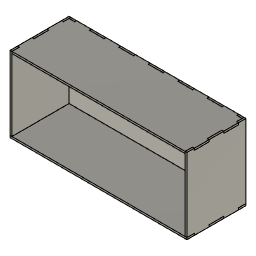
ShockBox 2.0 Enclosure v4 (Autodesk Fusion 360 design; units mm, degrees)
Autodesk Fusion 360 part; units mm, degrees
note: some values were not read from the file. Set by a fixed rule: which sketch regions a step uses.
sketch "Sketch1" plane through (0, 0, 0) normal (0, 1, 0) x (1, 0, 0)
  line L0 (0, 0) -> (304.8, 0)
  line L1 (304.8, 0) -> (304.8, -101.6)
  line L2 (304.8, -101.6) -> (0, -101.6)
  line L3 (0, -101.6) -> (0, 0)
  dimension "d1" = 304.8
  dimension "d2" = 101.6
  constraint horizontal L0
  constraint vertical L1
  constraint horizontal L2
  constraint vertical L3
  constraint coincident L0.start L3.end
  measures "d1" distance of L0.start L0.end
  measures "d2" distance of L0.end L1.end
extrude "Extrude1" add sketch "Sketch1" along normal blind 3.175 makes body 1 in component "Base"
sketch "Sketch2" plane through (0, 0, 0) normal (0, -1, 0) x (1, 0, 0)
  line L0 (304.8, 101.6) -> (0, 101.6)
  line L1 (0, 101.6) -> (0, 0)
  line L2 (0, 0) -> (304.8, 0)
  line L3 (304.8, 0) -> (304.8, 101.6)
  line L4 (0, 101.6) -> (0, 88.9)
  line L5 (0, 88.9) -> (3.175, 88.9)
  line L6 (3.175, 88.9) -> (3.175, 63.5)
  line L7 (3.175, 63.5) -> (0, 63.5)
  line L8 (0, 88.9) -> (0, 63.5)
  line L9 (0, 63.5) -> (0, 38.1)
  line L10 (0, 38.1) -> (3.175, 38.1)
  line L11 (3.175, 38.1) -> (3.175, 12.7)
  line L12 (3.175, 12.7) -> (0, 12.7)
  line L13 (0, 38.1) -> (0, 12.7)
  line L14 (0, 101.6) -> (12.7, 101.6)
  line L15 (12.7, 101.6) -> (12.7, 98.425)
  line L16 (12.7, 98.425) -> (38.1, 98.425)
  line L17 (38.1, 98.425) -> (38.1, 101.6)
  line L18 (38.1, 101.6) -> (12.7, 101.6)
  line L19 (38.1, 101.6) -> (63.5, 101.6)
  line L20 (63.5, 101.6) -> (63.5, 98.425)
  line L21 (63.5, 98.425) -> (88.9, 98.425)
  line L22 (88.9, 98.425) -> (88.9, 101.6)
  line L23 (88.9, 101.6) -> (63.5, 101.6)
  line L24 (88.9, 101.6) -> (114.3, 101.6)
  line L25 (114.3, 101.6) -> (114.3, 98.425)
  line L26 (114.3, 98.425) -> (139.7, 98.425)
  line L27 (139.7, 98.425) -> (139.7, 101.6)
  line L28 (139.7, 101.6) -> (114.3, 101.6)
  line L29 (139.7, 101.6) -> (165.1, 101.6)
  line L30 (165.1, 101.6) -> (165.1, 98.425)
  line L31 (165.1, 98.425) -> (190.5, 98.425)
  line L32 (190.5, 98.425) -> (190.5, 101.6)
  line L33 (190.5, 101.6) -> (165.1, 101.6)
  line L34 (190.5, 101.6) -> (215.9, 101.6)
  line L35 (215.9, 101.6) -> (215.9, 98.425)
  line L36 (215.9, 98.425) -> (241.3, 98.425)
  line L37 (241.3, 98.425) -> (241.3, 101.6)
  line L38 (215.9, 101.6) -> (241.3, 101.6)
  line L39 (241.3, 101.6) -> (266.7, 101.6)
  line L40 (266.7, 101.6) -> (266.7, 98.425)
  line L41 (266.7, 98.425) -> (292.1, 98.425)
  line L42 (292.1, 98.425) -> (292.1, 101.6)
  line L43 (292.1, 101.6) -> (266.7, 101.6)
  line L44 (304.8, 101.6) -> (304.8, 88.9)
  line L45 (304.8, 88.9) -> (301.625, 88.9)
  line L46 (301.625, 88.9) -> (301.625, 63.5)
  line L47 (301.625, 63.5) -> (304.8, 63.5)
  line L48 (304.8, 63.5) -> (304.8, 38.1)
  line L49 (304.8, 38.1) -> (301.625, 38.1)
  line L50 (301.625, 38.1) -> (301.625, 12.7)
  line L51 (301.625, 12.7) -> (304.8, 12.7)
  line L52 (304.8, 12.7) -> (304.8, 38.1)
  line L53 (304.8, 63.5) -> (304.8, 88.9)
  dimension "d7" = 12.7
  dimension "d8" = 3.175
  dimension "d9" = 25.4
  dimension "d10" = 25.4
  dimension "d11" = 3.175
  dimension "d12" = 25.4
  dimension "d13" = 12.7
  dimension "d14" = 3.175
  dimension "d15" = 25.4
  dimension "d16" = 25.4
  dimension "d17" = 3.175
  dimension "d18" = 25.4
  dimension "d19" = 25.4
  dimension "d20" = 3.175
  dimension "d21" = 25.4
  dimension "d22" = 25.4
  dimension "d23" = 3.175
  dimension "d24" = 25.4
  dimension "d25" = 25.4
  dimension "d26" = 25.4
  dimension "d27" = 25.4
  dimension "d28" = 25.4
  dimension "d29" = 12.7
  dimension "d30" = 3.175
  dimension "d31" = 25.4
  dimension "d32" = 25.4
  dimension "d33" = 3.175
  dimension "d34" = 25.4
  constraint coincident L0.end L1.start
  constraint perpendicular L0 L4
  constraint perpendicular L1 L5
  constraint perpendicular L5 L6
  constraint coincident L1 L7.end
  constraint perpendicular L1 L7
  constraint perpendicular L7 L9
  constraint perpendicular L1 L10
  constraint perpendicular L10 L11
  constraint coincident L1 L12.end
  constraint perpendicular L1 L12
  constraint perpendicular L4 L14
  constraint perpendicular L14 L15
  constraint perpendicular L15 L16
  constraint coincident L0 L17.end
  constraint perpendicular L0 L17
  constraint perpendicular L17 L19
  constraint perpendicular L19 L20
  constraint perpendicular L20 L21
  constraint coincident L0 L22.end
  constraint perpendicular L0 L22
  constraint perpendicular L22 L24
  constraint perpendicular L0 L25
  constraint perpendicular L25 L26
  constraint coincident L0 L27.end
  constraint perpendicular L0 L27
  constraint perpendicular L27 L29
  constraint perpendicular L29 L30
  constraint perpendicular L30 L31
  constraint coincident L0 L32.end
  constraint perpendicular L0 L32
  constraint perpendicular L32 L34
  constraint perpendicular L34 L35
  constraint perpendicular L35 L36
  constraint coincident L0 L37.end
  constraint perpendicular L0 L37
  constraint perpendicular L3 L39
  constraint perpendicular L39 L40
  constraint perpendicular L40 L41
  constraint coincident L0 L42.end
  constraint perpendicular L0 L42
  constraint coincident L0.start L3.end
  constraint perpendicular L0 L44
  constraint perpendicular L44 L45
  constraint perpendicular L45 L46
  constraint coincident L3 L47.end
  constraint perpendicular L3 L47
  constraint perpendicular L47 L48
  constraint perpendicular L48 L49
  constraint perpendicular L49 L50
  constraint coincident L3 L51.end
  constraint perpendicular L3 L51
  measures "d7" distance of L0.end L4.end
  measures "d8" distance of L4.end L5.end
  measures "d9" distance of L5.end L6.end
  measures "d10" distance of L7.end L9.end
  measures "d11" distance of L9.end L10.end
  measures "d12" distance of L10.end L11.end
  measures "d13" distance of L0.end L14.end
  measures "d14" distance of L14.end L15.end
  measures "d15" distance of L15.end L16.end
  measures "d16" distance of L17.end L19.end
  measures "d17" distance of L19.end L20.end
  measures "d18" distance of L20.end L21.end
  measures "d19" distance of L22.end L24.end
  measures "d20" distance of L24.end L25.end
  measures "d21" distance of L25.end L26.end
  measures "d22" distance of L27.end L29.end
  measures "d23" distance of L29.end L30.end
  measures "d24" distance of L30.end L31.end
  measures "d25" distance of L32.end L34.end
  measures "d26" distance of L35.end L36.end
  measures "d27" distance of L37.end L39.end
  measures "d28" distance of L40.end L41.end
  measures "d29" distance of L0.start L44.end
  measures "d30" distance of L44.end L45.end
  measures "d31" distance of L45.end L46.end
  measures "d32" distance of L47.end L48.end
  measures "d33" distance of L48.end L49.end
  measures "d34" distance of L49.end L50.end
extrude "Extrude2" cut sketch "Sketch2" against normal blind 53.34 contours L0 L40 L41 L42 L43 | L3 L45 L46 L47 L53 | L0 L35 L36 L37 L38 | L3 L49 L50 L51 L52 | L0 L30 L31 L32 L33 | L0 L25 L26 L27 L28 | L1 L10 L11 L12 L13 | L0 L20 L21 L22 L23 | L1 L5 L6 L7 L8 | L0 L15 L16 L17 L18 bodies 1 in component "Base"
sketch "Sketch3" plane through (0, 0, 0) normal (-1, 0, 0) x (0, -1, 0)
  line L0 (-3.175, 88.9) -> (0, 88.9)
  line L1 (0, 88.9) -> (0, 101.6)
  line L2 (0, 101.6) -> (-3.175, 101.6)
  line L3 (-3.175, 101.6) -> (-3.175, 88.9)
  line L4 (0, 101.6) -> (127, 101.6)
  line L5 (0, 0) -> (127, 0)
  line L6 (0, 101.6) -> (0, 88.9)
  line L7 (0, 88.9) -> (-3.175, 88.9)
  line L8 (-3.175, 88.9) -> (-3.175, 63.5)
  line L9 (-3.175, 63.5) -> (0, 63.5)
  line L10 (0, 63.5) -> (0, 38.1)
  line L11 (0, 38.1) -> (-3.175, 38.1)
  line L12 (-3.175, 38.1) -> (-3.175, 12.7)
  line L13 (-3.175, 12.7) -> (0, 12.7)
  line L14 (0, 12.7) -> (0, 0)
  line L15 (127, 0) -> (127, 12.7)
  line L16 (127, 12.7) -> (123.825, 12.7)
  line L17 (123.825, 12.7) -> (123.825, 38.1)
  line L18 (123.825, 38.1) -> (127, 38.1)
  line L19 (127, 38.1) -> (127, 63.5)
  line L20 (127, 63.5) -> (123.825, 63.5)
  line L21 (123.825, 63.5) -> (123.825, 88.9)
  line L22 (123.825, 88.9) -> (127, 88.9)
  line L23 (127, 88.9) -> (127, 101.6)
  dimension "d37" = 127
  dimension "d38" = 127
  dimension "d39" = 25.4
  dimension "d40" = 3.175
  dimension "d41" = 25.4
  dimension "d42" = 3.175
  dimension "d43" = 25.4
  dimension "d44" = 3.175
  dimension "d53" = 12.7
  dimension "d54" = 3.175
  dimension "d55" = 25.4
  dimension "d56" = 25.4
  dimension "d57" = 25.4
  constraint coincident L1.end L2.start
  constraint perpendicular L1 L4
  constraint coincident L5.start L14.end
  constraint horizontal L5
  constraint coincident L0.end L1.start
  constraint coincident L0.start L3.end
  constraint perpendicular L7 L8
  constraint perpendicular L8 L9
  constraint perpendicular L9 L10
  constraint perpendicular L10 L11
  constraint perpendicular L11 L12
  constraint perpendicular L12 L13
  constraint perpendicular L5 L15
  constraint perpendicular L15 L16
  constraint perpendicular L16 L17
  constraint perpendicular L17 L18
  constraint perpendicular L18 L19
  constraint perpendicular L19 L20
  constraint perpendicular L20 L21
  constraint perpendicular L21 L22
  constraint perpendicular L4 L23
  measures "d37" distance of L1.end L4.end
  measures "d38" distance of L5.start L5.end
  measures "d39" distance of L0.start L8.end
  measures "d40" distance of L8.end L9.end
  measures "d41" distance of L9.end L10.end
  measures "d42" distance of L10.end L11.end
  measures "d43" distance of L11.end L12.end
  measures "d44" distance of L12.end L13.end
  measures "d53" distance of L5.end L15.end
  measures "d54" distance of L15.end L16.end
  measures "d55" distance of L16.end L17.end
  measures "d56" distance of L18.end L19.end
  measures "d57" distance of L20.end L21.end
extrude "Extrude1'" add sketch "Sketch3" against normal blind 3.175 separate body contours L0 L1 L4 L5 L6 L7 L8 L9 L10 L11 L12 L13 L14 L15 L16 L17 L18 L19 L20 L21 L22 L23 makes body 2 in component "LeftWall"
sketch "FrontWallSketch" plane through (304.8, 0, 0) normal (1, 0, 0) x (0, 1, 0)
  line L0 (3.175, 63.5) -> (0, 63.5)
  line L1 (0, 63.5) -> (0, 38.1)
  line L2 (0, 38.1) -> (3.175, 38.1)
  line L3 (3.175, 38.1) -> (3.175, 63.5)
  line L4 (3.175, 12.7) -> (0, 12.7)
  line L5 (0, 12.7) -> (0, 0)
  line L6 (0, 0) -> (3.175, 0)
  line L7 (3.175, 0) -> (3.175, 12.7)
  line L8 (0, 88.9) -> (3.175, 88.9)
  line L9 (3.175, 88.9) -> (3.175, 101.6)
  line L10 (3.175, 101.6) -> (0, 101.6)
  line L11 (0, 101.6) -> (0, 88.9)
  line L12 (0, 0) -> (0, 12.7)
  line L13 (0, 12.7) -> (3.175, 12.7)
  line L14 (3.175, 12.7) -> (3.175, 38.1)
  line L15 (3.175, 38.1) -> (0, 38.1)
  line L16 (0, 38.1) -> (0, 63.5)
  line L17 (0, 63.5) -> (3.175, 63.5)
  line L18 (3.175, 63.5) -> (3.175, 88.9)
  line L19 (3.175, 88.9) -> (0, 88.9)
  line L20 (0, 88.9) -> (0, 101.6)
  line L21 (0, 101.6) -> (-127, 101.6)
  line L22 (0, 0) -> (-127, 0)
  line L23 (0, 88.9) -> (0, 101.6)
  line L24 (0, 101.6) -> (-127, 101.6)
  line L25 (-127, 101.6) -> (-127, 88.9)
  line L26 (-127, 88.9) -> (-123.825, 88.9)
  line L27 (-123.825, 88.9) -> (-123.825, 63.5)
  line L28 (-123.825, 63.5) -> (-127, 63.5)
  line L29 (-127, 63.5) -> (-127, 38.1)
  line L30 (-127, 38.1) -> (-123.825, 38.1)
  line L31 (-123.825, 38.1) -> (-123.825, 12.7)
  line L32 (-123.825, 12.7) -> (-127, 12.7)
  line L33 (-127, 12.7) -> (-127, 0)
  line L34 (-127, 0) -> (0, 0)
  line L35 (0, 0) -> (0, 12.7)
  line L36 (0, 12.7) -> (3.175, 12.7)
  line L37 (3.175, 12.7) -> (3.175, 38.1)
  line L38 (3.175, 38.1) -> (0, 38.1)
  line L39 (0, 38.1) -> (0, 63.5)
  line L40 (0, 63.5) -> (3.175, 63.5)
  line L41 (3.175, 63.5) -> (3.175, 88.9)
  line L42 (3.175, 88.9) -> (0, 88.9)
  line L43 (-127, 0) -> (-127, 12.7)
  line L44 (-127, 12.7) -> (-123.825, 12.7)
  line L45 (-123.825, 12.7) -> (-123.825, 38.1)
  line L46 (-127, 38.1) -> (-123.825, 38.1)
  line L47 (-127, 38.1) -> (-127, 63.5)
  line L48 (-127, 63.5) -> (-123.825, 63.5)
  line L49 (-123.825, 63.5) -> (-123.825, 88.9)
  line L50 (-127, 88.9) -> (-123.825, 88.9)
  line L51 (-127, 88.9) -> (-127, 101.6)
  dimension "d47" = 127
  dimension "d48" = 127
  constraint coincident L5.end L6.start
  constraint coincident L4.end L5.start
  constraint coincident L4.start L7.end
  constraint coincident L2.end L3.start
  constraint coincident L1.end L2.start
  constraint coincident L0.end L1.start
  constraint coincident L0.start L3.end
  constraint coincident L8.end L9.start
  constraint coincident L8.start L11.end
  constraint coincident L10.end L11.start
  constraint perpendicular L20 L21
  constraint perpendicular L12 L22
  constraint coincident L32.end L33.start
  constraint coincident L31.end L32.start
  constraint coincident L30.end L31.start
  constraint coincident L29.end L30.start
  constraint coincident L28.end L29.start
  constraint coincident L27.end L28.start
  constraint coincident L26.end L27.start
  constraint coincident L25.end L26.start
  constraint coincident L21.end L24.end
  measures "d47" distance of L10.end L21.end
  measures "d48" distance of L5.end L22.end
extrude "Extrude1''" add sketch "FrontWallSketch" against normal blind 3.175 separate body contours L0 L1 L2 L4 L5 L8 L11 L12 L13 L14 L15 L16 L17 L18 L19 L20 L21 L22 L23 L24 L25 L26 L27 L28 L29 L30 L31 L32 L33 L34 L35 L36 L37 L38 L39 L40 L41 L42 L43 L44 L45 L46 L47 L48 L49 L50 L51 makes body 3 in component "RightWall"
sketch "Sketch5" plane through (0, 0, 101.6) normal (0, 0, 1) x (-1, 0, 0)
  line L0 (-266.7, 0) -> (-266.7, -3.175)
  line L1 (-266.7, -3.175) -> (-241.3, -3.175)
  line L2 (-241.3, -3.175) -> (-241.3, 0)
  line L3 (-241.3, 0) -> (-266.7, 0)
  line L4 (-304.8, 127) -> (-304.8, 0)
  line L5 (-304.8, 0) -> (-301.625, 0)
  line L6 (-301.625, 0) -> (-301.625, 127)
  line L7 (-292.1, -3.175) -> (-292.1, 0)
  line L8 (-292.1, 0) -> (-304.8, 0)
  line L9 (-304.8, 0) -> (-304.8, -3.175)
  line L10 (-304.8, -3.175) -> (-292.1, -3.175)
  line L11 (-215.9, 0) -> (-215.9, -3.175)
  line L12 (-215.9, -3.175) -> (-190.5, -3.175)
  line L13 (-190.5, -3.175) -> (-190.5, 0)
  line L14 (-190.5, 0) -> (-215.9, 0)
  line L15 (-139.7, -3.175) -> (-139.7, 0)
  line L16 (-139.7, 0) -> (-165.1, 0)
  line L17 (-165.1, 0) -> (-165.1, -3.175)
  line L18 (-165.1, -3.175) -> (-139.7, -3.175)
  line L19 (-88.9, -3.175) -> (-88.9, 0)
  line L20 (-88.9, 0) -> (-114.3, 0)
  line L21 (-114.3, 0) -> (-114.3, -3.175)
  line L22 (-114.3, -3.175) -> (-88.9, -3.175)
  line L23 (-63.5, 0) -> (-63.5, -3.175)
  line L24 (-63.5, -3.175) -> (-38.1, -3.175)
  line L25 (-38.1, -3.175) -> (-38.1, 0)
  line L26 (-38.1, 0) -> (-63.5, 0)
  line L27 (-12.7, 0) -> (-12.7, -3.175)
  line L28 (-12.7, -3.175) -> (0, -3.175)
  line L29 (0, -3.175) -> (0, 0)
  line L30 (0, 0) -> (-12.7, 0)
  line L31 (0, 0) -> (0, 127)
  line L32 (-3.175, 127) -> (-3.175, 0)
  line L33 (-3.175, 0) -> (0, 0)
  line L34 (-301.625, 0) -> (-292.1, 0)
  line L35 (-292.1, 0) -> (-292.1, -3.175)
  line L36 (-292.1, -3.175) -> (-266.7, -3.175)
  line L37 (-266.7, -3.175) -> (-266.7, 0)
  line L38 (-266.7, 0) -> (-241.3, 0)
  line L39 (-241.3, 0) -> (-241.3, -3.175)
  line L40 (-215.9, -3.175) -> (-241.3, -3.175)
  line L41 (-215.9, 0) -> (-215.9, -3.175)
  line L42 (-215.9, 0) -> (-190.5, 0)
  line L43 (-190.5, 0) -> (-190.5, -3.175)
  line L44 (-190.5, -3.175) -> (-165.1, -3.175)
  line L45 (-165.1, -3.175) -> (-165.1, 0)
  line L46 (-165.1, 0) -> (-139.7, 0)
  line L47 (-139.7, 0) -> (-139.7, -3.175)
  line L48 (-139.7, -3.175) -> (-114.3, -3.175)
  line L49 (-114.3, -3.175) -> (-114.3, 0)
  line L50 (-114.3, 0) -> (-88.9, 0)
  line L51 (-88.9, 0) -> (-88.9, -3.175)
  line L52 (-88.9, -3.175) -> (-63.5, -3.175)
  line L53 (-63.5, -3.175) -> (-63.5, 0)
  line L54 (-63.5, 0) -> (-38.1, 0)
  line L55 (-38.1, 0) -> (-38.1, -3.175)
  line L56 (-12.7, -3.175) -> (-38.1, -3.175)
  line L57 (-12.7, -3.175) -> (-12.7, 0)
  line L58 (-12.7, 0) -> (-3.175, 0)
  line L59 (-301.625, 127) -> (-301.625, 0)
  line L60 (-3.175, 127) -> (-3.175, 0)
  line L61 (0, 127) -> (-3.175, 127)
  line L62 (-301.625, 127) -> (-304.8, 127)
  line L63 (-3.175, 127) -> (-12.7, 127)
  line L64 (-12.7, 127) -> (-12.7, 123.825)
  line L65 (-12.7, 123.825) -> (-38.1, 123.825)
  line L66 (-38.1, 123.825) -> (-38.1, 127)
  line L67 (-38.1, 127) -> (-63.5, 127)
  line L68 (-63.5, 127) -> (-63.5, 123.825)
  line L69 (-63.5, 123.825) -> (-88.9, 123.825)
  line L70 (-88.9, 123.825) -> (-88.9, 127)
  line L71 (-88.9, 127) -> (-114.3, 127)
  line L72 (-114.3, 127) -> (-114.3, 123.825)
  line L73 (-114.3, 123.825) -> (-139.7, 123.825)
  line L74 (-139.7, 123.825) -> (-139.7, 127)
  line L75 (-139.7, 127) -> (-165.1, 127)
  line L76 (-165.1, 127) -> (-165.1, 123.825)
  line L77 (-165.1, 123.825) -> (-190.5, 123.825)
  line L78 (-190.5, 123.825) -> (-190.5, 127)
  line L79 (-190.5, 127) -> (-215.9, 127)
  line L80 (-215.9, 127) -> (-215.9, 123.825)
  line L81 (-215.9, 123.825) -> (-241.3, 123.825)
  line L82 (-241.3, 123.825) -> (-241.3, 127)
  line L83 (-241.3, 127) -> (-266.7, 127)
  line L84 (-266.7, 127) -> (-266.7, 123.825)
  line L85 (-266.7, 123.825) -> (-292.1, 123.825)
  line L86 (-292.1, 123.825) -> (-292.1, 127)
  line L87 (-292.1, 127) -> (-301.625, 127)
  dimension "d58" = 9.525
  dimension "d59" = 3.175
  dimension "d60" = 25.4
  dimension "d61" = 3.175
  dimension "d62" = 25.4
  dimension "d63" = 3.175
  dimension "d64" = 25.4
  dimension "d65" = 3.175
  dimension "d66" = 25.4
  dimension "d67" = 3.175
  dimension "d68" = 25.4
  dimension "d69" = 3.175
  dimension "d70" = 25.4
  dimension "d71" = 3.175
  dimension "d72" = 25.4
  dimension "d73" = 3.175
  dimension "d74" = 25.4
  dimension "d75" = 3.175
  dimension "d76" = 25.4
  dimension "d77" = 3.175
  dimension "d78" = 25.4
  dimension "d79" = 3.175
  dimension "d80" = 25.4
  dimension "d81" = 3.175
  constraint coincident L5.end L6.start
  constraint coincident L7.end L8.start
  constraint coincident L7.start L10.end
  constraint coincident L0.end L1.start
  constraint coincident L0.start L3.end
  constraint coincident L2.end L3.start
  constraint coincident L1.end L2.start
  constraint coincident L11.end L12.start
  constraint coincident L11.start L14.end
  constraint coincident L13.end L14.start
  constraint coincident L12.end L13.start
  constraint coincident L17.end L18.start
  constraint coincident L16.end L17.start
  constraint coincident L15.end L16.start
  constraint coincident L15.start L18.end
  constraint coincident L21.end L22.start
  constraint coincident L20.end L21.start
  constraint coincident L19.end L20.start
  constraint coincident L19.start L22.end
  constraint coincident L23.end L24.start
  constraint coincident L23.start L26.end
  constraint coincident L25.end L26.start
  constraint coincident L24.end L25.start
  constraint coincident L27.end L28.start
  constraint coincident L27.start L30.end
  constraint coincident L32.end L33.start
  constraint coincident L6.end L59.start
  constraint coincident L32.start L60.start
  constraint perpendicular L60 L63
  constraint perpendicular L63 L64
  constraint perpendicular L64 L65
  constraint perpendicular L65 L66
  constraint perpendicular L66 L67
  constraint perpendicular L67 L68
  constraint perpendicular L68 L69
  constraint perpendicular L69 L70
  constraint perpendicular L70 L71
  constraint perpendicular L71 L72
  constraint perpendicular L72 L73
  constraint perpendicular L73 L74
  constraint perpendicular L74 L75
  constraint perpendicular L75 L76
  constraint perpendicular L76 L77
  constraint perpendicular L77 L78
  constraint perpendicular L78 L79
  constraint perpendicular L79 L80
  constraint perpendicular L80 L81
  constraint perpendicular L81 L82
  constraint perpendicular L82 L83
  constraint perpendicular L83 L84
  constraint perpendicular L84 L85
  constraint perpendicular L85 L86
  measures "d58" distance of L32.start L63.end
  measures "d59" distance of L63.end L64.end
  measures "d60" distance of L64.end L65.end
  measures "d61" distance of L65.end L66.end
  measures "d62" distance of L66.end L67.end
  measures "d63" distance of L67.end L68.end
  measures "d64" distance of L68.end L69.end
  measures "d65" distance of L69.end L70.end
  measures "d66" distance of L70.end L71.end
  measures "d67" distance of L71.end L72.end
  measures "d68" distance of L72.end L73.end
  measures "d69" distance of L73.end L74.end
  measures "d70" distance of L74.end L75.end
  measures "d71" distance of L75.end L76.end
  measures "d72" distance of L76.end L77.end
  measures "d73" distance of L77.end L78.end
  measures "d74" distance of L78.end L79.end
  measures "d75" distance of L79.end L80.end
  measures "d76" distance of L80.end L81.end
  measures "d77" distance of L81.end L82.end
  measures "d78" distance of L82.end L83.end
  measures "d79" distance of L83.end L84.end
  measures "d80" distance of L84.end L85.end
  measures "d81" distance of L85.end L86.end
extrude "Extrude1'''" add sketch "Sketch5" against normal blind 3.175 separate body contours L0 L2 L3 L6 L7 L8 L11 L13 L14 L15 L16 L17 L19 L20 L21 L23 L25 L26 L27 L30 L32 L34 L35 L36 L37 L38 L39 L40 L41 L42 L43 L44 L45 L46 L47 L48 L49 L50 L51 L52 L53 L54 L55 L56 L57 L58 L59 L60 L63 L64 L65 L66 L67 L68 L69 L70 L71 L72 L73 L74 L75 L76 L77 L78 L79 L80 L81 L82 L83 L84 L85 L86 L87 makes body 4 in component "FrontWall"
sketch "TopSketch" plane through (0, -127, 0) normal (0, -1, 0) x (1, 0, 0)
  line L0 (0, 12.7) -> (0, 0)
  line L1 (0, 0) -> (3.175, 0)
  line L2 (3.175, 0) -> (3.175, 12.7)
  line L3 (3.175, 12.7) -> (0, 12.7)
  line L4 (0, 63.5) -> (0, 38.1)
  line L5 (0, 38.1) -> (3.175, 38.1)
  line L6 (3.175, 38.1) -> (3.175, 63.5)
  line L7 (3.175, 63.5) -> (0, 63.5)
  line L8 (0, 101.6) -> (0, 88.9)
  line L9 (0, 88.9) -> (3.175, 88.9)
  line L10 (3.175, 88.9) -> (3.175, 101.6)
  line L11 (3.175, 101.6) -> (0, 101.6)
  line L12 (12.7, 101.6) -> (3.175, 101.6)
  line L13 (3.175, 101.6) -> (3.175, 98.425)
  line L14 (3.175, 98.425) -> (12.7, 98.425)
  line L15 (12.7, 98.425) -> (12.7, 101.6)
  line L16 (63.5, 101.6) -> (38.1, 101.6)
  line L17 (38.1, 101.6) -> (38.1, 98.425)
  line L18 (38.1, 98.425) -> (63.5, 98.425)
  line L19 (63.5, 98.425) -> (63.5, 101.6)
  line L20 (114.3, 101.6) -> (88.9, 101.6)
  line L21 (88.9, 101.6) -> (88.9, 98.425)
  line L22 (88.9, 98.425) -> (114.3, 98.425)
  line L23 (114.3, 98.425) -> (114.3, 101.6)
  line L24 (165.1, 101.6) -> (139.7, 101.6)
  line L25 (139.7, 101.6) -> (139.7, 98.425)
  line L26 (139.7, 98.425) -> (165.1, 98.425)
  line L27 (165.1, 98.425) -> (165.1, 101.6)
  line L28 (215.9, 101.6) -> (190.5, 101.6)
  line L29 (190.5, 101.6) -> (190.5, 98.425)
  line L30 (190.5, 98.425) -> (215.9, 98.425)
  line L31 (215.9, 98.425) -> (215.9, 101.6)
  line L32 (266.7, 101.6) -> (241.3, 101.6)
  line L33 (241.3, 101.6) -> (241.3, 98.425)
  line L34 (241.3, 98.425) -> (266.7, 98.425)
  line L35 (266.7, 98.425) -> (266.7, 101.6)
  line L36 (301.625, 101.6) -> (292.1, 101.6)
  line L37 (292.1, 101.6) -> (292.1, 98.425)
  line L38 (292.1, 98.425) -> (301.625, 98.425)
  line L39 (301.625, 98.425) -> (301.625, 101.6)
  line L40 (304.8, 88.9) -> (304.8, 101.6)
  line L41 (304.8, 101.6) -> (301.625, 101.6)
  line L42 (301.625, 101.6) -> (301.625, 88.9)
  line L43 (301.625, 88.9) -> (304.8, 88.9)
  line L44 (304.8, 38.1) -> (304.8, 63.5)
  line L45 (304.8, 63.5) -> (301.625, 63.5)
  line L46 (301.625, 63.5) -> (301.625, 38.1)
  line L47 (301.625, 38.1) -> (304.8, 38.1)
  line L48 (304.8, 0) -> (304.8, 12.7)
  line L49 (304.8, 12.7) -> (301.625, 12.7)
  line L50 (301.625, 12.7) -> (301.625, 0)
  line L51 (301.625, 0) -> (304.8, 0)
  line L52 (0, 12.7) -> (0, 38.1)
  line L53 (0, 12.7) -> (3.175, 12.7)
  line L54 (3.175, 12.7) -> (3.175, 0)
  line L55 (3.175, 0) -> (301.625, 0)
  line L56 (0, 38.1) -> (3.175, 38.1)
  line L57 (3.175, 38.1) -> (3.175, 63.5)
  line L58 (3.175, 63.5) -> (0, 63.5)
  line L59 (0, 63.5) -> (0, 88.9)
  line L60 (0, 88.9) -> (3.175, 88.9)
  line L61 (3.175, 88.9) -> (3.175, 98.425)
  line L62 (3.175, 98.425) -> (12.7, 98.425)
  line L63 (12.7, 98.425) -> (12.7, 101.6)
  line L64 (12.7, 101.6) -> (38.1, 101.6)
  line L65 (38.1, 101.6) -> (38.1, 98.425)
  line L66 (38.1, 98.425) -> (63.5, 98.425)
  line L67 (63.5, 98.425) -> (63.5, 101.6)
  line L68 (63.5, 101.6) -> (88.9, 101.6)
  line L69 (88.9, 101.6) -> (88.9, 98.425)
  line L70 (88.9, 98.425) -> (114.3, 98.425)
  line L71 (114.3, 98.425) -> (114.3, 101.6)
  line L72 (114.3, 101.6) -> (139.7, 101.6)
  line L73 (139.7, 101.6) -> (139.7, 98.425)
  line L74 (139.7, 98.425) -> (165.1, 98.425)
  line L75 (165.1, 98.425) -> (165.1, 101.6)
  line L76 (165.1, 101.6) -> (190.5, 101.6)
  line L77 (190.5, 98.425) -> (190.5, 101.6)
  line L78 (190.5, 98.425) -> (215.9, 98.425)
  line L79 (215.9, 98.425) -> (215.9, 101.6)
  line L80 (241.3, 101.6) -> (215.9, 101.6)
  line L81 (241.3, 101.6) -> (241.3, 98.425)
  line L82 (241.3, 98.425) -> (266.7, 98.425)
  line L83 (266.7, 98.425) -> (266.7, 101.6)
  line L84 (266.7, 101.6) -> (292.1, 101.6)
  line L85 (292.1, 101.6) -> (292.1, 98.425)
  line L86 (292.1, 98.425) -> (301.625, 98.425)
  line L87 (301.625, 98.425) -> (301.625, 88.9)
  line L88 (301.625, 88.9) -> (304.8, 88.9)
  line L89 (304.8, 88.9) -> (304.8, 63.5)
  line L90 (304.8, 63.5) -> (301.625, 63.5)
  line L91 (301.625, 63.5) -> (301.625, 38.1)
  line L92 (301.625, 38.1) -> (304.8, 38.1)
  line L93 (304.8, 38.1) -> (304.8, 12.7)
  line L94 (304.8, 12.7) -> (301.625, 12.7)
  line L95 (301.625, 12.7) -> (301.625, 0)
  constraint coincident L0.start L3.end
  constraint coincident L4.end L5.start
  constraint coincident L2.end L3.start
  constraint coincident L1.end L2.start
  constraint coincident L50.end L51.start
  constraint coincident L5.end L6.start
  constraint coincident L6.end L7.start
  constraint coincident L4.start L7.end
  constraint coincident L8.end L9.start
  constraint coincident L9.end L10.start
  constraint coincident L13.end L14.start
  constraint coincident L14.end L15.start
  constraint coincident L12.start L15.end
  constraint coincident L16.end L17.start
  constraint coincident L17.end L18.start
  constraint coincident L18.end L19.start
  constraint coincident L16.start L19.end
  constraint coincident L20.end L21.start
  constraint coincident L21.end L22.start
  constraint coincident L22.end L23.start
  constraint coincident L20.start L23.end
  constraint coincident L24.end L25.start
  constraint coincident L25.end L26.start
  constraint coincident L26.end L27.start
  constraint coincident L24.start L27.end
  constraint coincident L28.end L29.start
  constraint coincident L29.end L30.start
  constraint coincident L30.end L31.start
  constraint coincident L28.start L31.end
  constraint coincident L32.end L33.start
  constraint coincident L33.end L34.start
  constraint coincident L34.end L35.start
  constraint coincident L32.start L35.end
  constraint coincident L36.end L37.start
  constraint coincident L37.end L38.start
  constraint coincident L38.end L39.start
  constraint coincident L42.end L43.start
  constraint coincident L40.start L43.end
  constraint coincident L44.end L45.start
  constraint coincident L45.end L46.start
  constraint coincident L46.end L47.start
  constraint perpendicular L91 L92
  constraint coincident L48.end L49.start
  constraint perpendicular L92 L93
  constraint coincident L49.end L50.start
extrude "Extrude1''''" add sketch "TopSketch" against normal blind 3.175 separate body contours L2 L3 L5 L6 L7 L9 L10 L14 L15 L17 L18 L19 L21 L22 L23 L25 L26 L27 L29 L30 L31 L33 L34 L35 L37 L38 L42 L43 L45 L46 L47 L49 L50 L52 L53 L54 L55 L56 L57 L58 L59 L60 L61 L62 L63 L64 L65 L66 L67 L68 L69 L70 L71 L72 L73 L74 L75 L76 L77 L78 L79 L80 L81 L82 L83 L84 L85 L86 L87 L88 L89 L90 L91 L92 L93 L94 L95 makes body 5 in component "Top"
sketch "BottomSketch" plane through (0, 3.175, 0) normal (0, 1, 0) x (-1, 0, 0)
  line L0 (-266.7, 101.6) -> (-266.7, 98.425)
  line L1 (-266.7, 98.425) -> (-292.1, 98.425)
  line L2 (-292.1, 98.425) -> (-292.1, 101.6)
  line L3 (-292.1, 101.6) -> (-304.8, 101.6)
  line L4 (-304.8, 101.6) -> (-304.8, 88.9)
  line L5 (-304.8, 88.9) -> (-301.625, 88.9)
  line L6 (-301.625, 88.9) -> (-301.625, 63.5)
  line L7 (-301.625, 63.5) -> (-304.8, 63.5)
  line L8 (-304.8, 63.5) -> (-304.8, 38.1)
  line L9 (-304.8, 38.1) -> (-301.625, 38.1)
  line L10 (-301.625, 38.1) -> (-301.625, 12.7)
  line L11 (-301.625, 12.7) -> (-304.8, 12.7)
  line L12 (-304.8, 12.7) -> (-304.8, 0)
  line L13 (-304.8, 0) -> (0, 0)
  line L14 (0, 0) -> (0, 12.7)
  line L15 (0, 12.7) -> (-3.175, 12.7)
  line L16 (-3.175, 12.7) -> (-3.175, 38.1)
  line L17 (-3.175, 38.1) -> (0, 38.1)
  line L18 (0, 38.1) -> (0, 63.5)
  line L19 (0, 63.5) -> (-3.175, 63.5)
  line L20 (-3.175, 63.5) -> (-3.175, 88.9)
  line L21 (-3.175, 88.9) -> (0, 88.9)
  line L22 (0, 88.9) -> (0, 101.6)
  line L23 (0, 101.6) -> (-12.7, 101.6)
  line L24 (-12.7, 101.6) -> (-12.7, 98.425)
  line L25 (-12.7, 98.425) -> (-38.1, 98.425)
  line L26 (-38.1, 98.425) -> (-38.1, 101.6)
  line L27 (-38.1, 101.6) -> (-63.5, 101.6)
  line L28 (-63.5, 101.6) -> (-63.5, 98.425)
  line L29 (-63.5, 98.425) -> (-88.9, 98.425)
  line L30 (-88.9, 98.425) -> (-88.9, 101.6)
  line L31 (-88.9, 101.6) -> (-114.3, 101.6)
  line L32 (-114.3, 101.6) -> (-114.3, 98.425)
  line L33 (-114.3, 98.425) -> (-139.7, 98.425)
  line L34 (-139.7, 98.425) -> (-139.7, 101.6)
  line L35 (-139.7, 101.6) -> (-165.1, 101.6)
  line L36 (-165.1, 101.6) -> (-165.1, 98.425)
  line L37 (-165.1, 98.425) -> (-190.5, 98.425)
  line L38 (-190.5, 98.425) -> (-190.5, 101.6)
  line L39 (-190.5, 101.6) -> (-215.9, 101.6)
  line L40 (-215.9, 101.6) -> (-215.9, 98.425)
  line L41 (-215.9, 98.425) -> (-241.3, 98.425)
  line L42 (-241.3, 98.425) -> (-241.3, 101.6)
  line L43 (-241.3, 101.6) -> (-266.7, 101.6)
component "Base" placed x (1, 0, 0) y (0, 1, 0) z (0, 0, 1) at (0, 0, 0)
component "LeftWall" placed x (1, 0, 0) y (0, 1, 0) z (0, 0, 1) at (0, 0, 0)
component "RightWall" placed x (1, 0, 0) y (0, 1, 0) z (0, 0, 1) at (0, 0, 0)
component "FrontWall" placed x (1, 0, 0) y (0, 1, 0) z (0, 0, 1) at (0, 0, 0)
component "Top" placed x (1, 0, 0) y (0, 1, 0) z (0, 0, 1) at (0, 0, 0)
